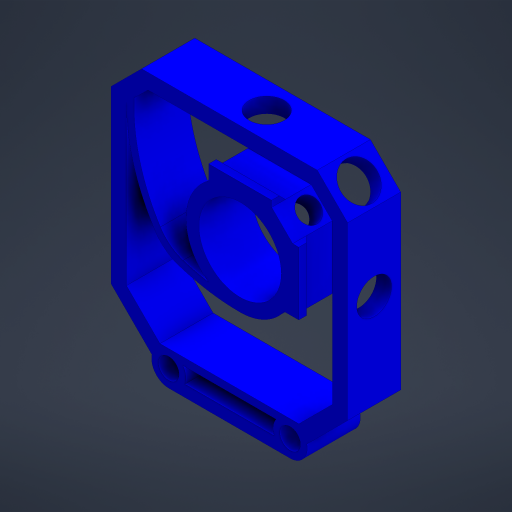
# Autodesk Inventor part: SM05 Lense Holder (V5)
Saved by Autodesk Inventor 2023.4 (Build 274418000, 418)
## iProperties
Created: 2022-07-25
Part Number: SM05 Lense Holder (V5)
Material: Generic
Document SubType Name: Modeling
Designer: xSibe
Density: 1 g/cm^3
Appearance: Plastic Blue
Author: xSibe
Autodesk Inventor part; units mm, degrees
ref_plane "YZ Plane" through (0, 0, 0) normal (1, 0, 0) x (0, 1, 0)
ref_plane "XZ Plane" through (0, 0, 0) normal (0, 1, 0) x (-1, 0, 0)
sketch "Sketch1" plane through (0, 0, 0) normal (0, 0, 1) x (1, 0, 0)
  circle A0 centre (139.6, 3.85) radius 2.8125
  circle A1 centre (159.6, 3.85) radius 2.8125
  line L0 (159.6, 1.0375) -> (139.6, 1.0375)
  line L1 (132.55, 24.9) -> (166.65, 24.9)
  line L2 (149.6, 24.9) -> (151.367767, 26.667767)
  line L3 (149.6, 24.9) -> (152.1, 24.9) construction
  circle A2 centre (151.367767, 26.667767) radius 6.78375
  circle A3 centre (151.367767, 26.667767) radius 6.10875
  circle A4 centre (151.367767, 26.667767) radius 8.90875
  line L4 (151.367767, 26.667767) -> (151.367767, 35.576517)
  line L5 (151.367767, 35.576517) -> (151.367767, 35.076517)
  line L6 (146.180267, 33.826517) -> (156.555267, 33.826517)
  line L7 (156.555267, 33.826517) -> (156.555267, 36.326517)
  line L8 (156.555267, 36.326517) -> (146.180267, 36.326517)
  line L9 (146.180267, 36.326517) -> (146.180267, 33.826517)
  line L10 (146.180267, 33.826517) -> (156.555267, 36.326517) construction
  line L11 (156.555267, 33.826517) -> (146.180267, 36.326517) construction
  line L12 (151.367767, 26.667767) -> (157.667204, 32.967204)
  line L13 (157.667204, 32.967204) -> (157.225263, 32.525263)
  line L14 (160.05369, 31.818156) -> (156.518156, 35.35369)
  line L15 (156.518156, 35.35369) -> (154.396836, 33.23237)
  line L16 (154.396836, 33.23237) -> (157.93237, 29.696836)
  line L17 (157.93237, 29.696836) -> (160.05369, 31.818156)
  line L18 (160.05369, 31.818156) -> (154.396836, 33.23237) construction
  line L19 (156.518156, 35.35369) -> (157.93237, 29.696836) construction
  line L20 (160.05369, 31.818156) -> (165.05369, 31.818156) construction
  line L21 (158.526517, 21.480267) -> (158.526517, 31.855267)
  line L22 (158.526517, 31.855267) -> (161.026517, 31.855267)
  line L23 (161.026517, 31.855267) -> (161.026517, 21.480267)
  line L24 (161.026517, 21.480267) -> (158.526517, 21.480267)
  line L25 (151.367767, 35.576517) -> (151.367767, 37.576517)
  line L26 (161.026517, 26.667767) -> (163.026517, 26.667767)
  line L27 (139.382233, 5.432233) -> (159.817767, 5.432233)
  line L28 (169.067767, 14.682233) -> (169.067767, 39.367767)
  line L29 (164.067767, 44.367767) -> (135.132233, 44.367767)
  line L30 (130.132233, 39.367767) -> (130.132233, 14.682233)
  line L31 (130.132233, 5.432233) -> (169.067767, 44.367767) construction
  line L32 (169.067767, 5.432233) -> (130.132233, 44.367767) construction
  line L33 (139.382233, 5.432233) -> (130.132233, 14.682233)
  line L34 (159.817767, 5.432233) -> (169.067767, 14.682233)
  line L35 (164.067767, 44.367767) -> (169.067767, 39.367767)
  line L36 (135.132233, 44.367767) -> (130.132233, 39.367767)
  line L37 (134.096699, 46.867767) -> (127.632233, 40.403301)
  line L38 (127.632233, 40.403301) -> (127.632233, 13.646699)
  line L39 (127.632233, 13.646699) -> (138.346699, 2.932233)
  line L40 (138.346699, 2.932233) -> (160.853301, 2.932233)
  line L41 (160.853301, 2.932233) -> (171.567767, 13.646699)
  line L42 (171.567767, 13.646699) -> (171.567767, 40.403301)
  line L43 (171.567767, 40.403301) -> (165.103301, 46.867767)
  line L44 (165.103301, 46.867767) -> (134.096699, 46.867767)
  line L45 (136.167767, 41.867767) -> (132.632233, 38.332233)
  line L46 (132.632233, 38.332233) -> (132.632233, 15.717767)
  line L47 (132.632233, 15.717767) -> (140.417767, 7.932233)
  line L48 (140.417767, 7.932233) -> (158.782233, 7.932233)
  line L49 (158.782233, 7.932233) -> (166.567767, 15.717767)
  line L50 (166.567767, 15.717767) -> (166.567767, 38.332233)
  line L51 (166.567767, 38.332233) -> (163.032233, 41.867767)
  line L52 (163.032233, 41.867767) -> (136.167767, 41.867767)
  line L53 (130.132233, 14.682233) -> (130.132233, 11.146699)
  line L54 (169.067767, 14.682233) -> (169.067767, 11.146699)
  circle A5 centre (139.6, 3.85) radius 1.705
  circle A6 centre (159.6, 3.85) radius 1.705
  line L55 (151.367767, 17.759017) -> (138.867767, 17.759017)
  line L56 (138.867767, 17.759017) -> (138.867767, 20.259017)
  arc A7 (138.867767, 20.259017) -> (151.367767, 17.759017) centre (151.367767, 50.259017) ccw
  arc A8 (132.632233, 38.332233) -> (138.867767, 20.259017) centre (161.941914, 38.332233) ccw
  arc A9 (133.911405, 39.611405) -> (139.651699, 21.288407) centre (161.941914, 38.332233) ccw
  arc A10 (139.651699, 21.288407) -> (146.148582, 19.447938) centre (151.367767, 50.259017) ccw
  line L57 (138.867767, 20.259017) -> (137.411533, 22.291105)
  line L58 (139.651699, 21.288407) -> (138.223144, 23.340048)
  arc A11 (137.411533, 22.291105) -> (141.173712, 19.399152) centre (143.428852, 26.226005) ccw
  arc A12 (138.223144, 23.340048) -> (141.966404, 20.45672) centre (144.034782, 27.013474) ccw
  line L59 (132.55, 7.7) -> (132.55, 42.1)
  line L60 (166.65, 7.7) -> (166.65, 42.1)
  circle A13 centre (139.6, 3.85) radius 1.5625
  circle A14 centre (159.6, 3.85) radius 1.5625
  line L61 (138.151966, 6.6625) -> (161.048034, 6.6625)
  line L62 (139.6, 5.555) -> (159.6, 5.555)
  line L63 (139.6, 2.145) -> (159.6, 2.145)
  line L64 (132.632233, 15.717767) -> (132.632233, 12.182233)
  line L65 (166.567767, 15.717767) -> (166.567767, 12.182233)
  point P0 (156.941455, 2.932233)
  point P1 (142.258545, 2.932233)
  point P2 (138.414176, 6.40029)
  point P3 (160.785824, 6.40029)
  point P4 (146.180267, 33.910396)
  point P5 (158.610396, 21.480267)
  point P6 (158.610396, 31.855267)
  point P7 (159.181848, 30.946314)
  point P8 (155.646314, 34.481848)
  point P9 (156.555267, 33.910396)
  point P10 (162.351875, 4.430808)
  point P11 (136.848125, 4.430808)
  point P12 (154.990983, 33.826517)
  point P13 (-2.842005, 34.542767)
  point P14 (9.642767, 22.057995)
  point P15 (158.526517, 30.290983)
  point P16 (10.676517, 26.667767)
  point P17 (160.016579, 31.855267)
  point P18 (9.642767, 31.277539)
  point P19 (6.377539, 34.542767)
  point P20 (1.767767, 35.576517)
  point P21 (156.555267, 35.316579)
  point P22 (8.067204, 32.967204)
  point P23 (166.567767, 24.9)
  point P24 (132.632233, 24.9)
  point P25 (160.099366, 24.9)
  point P26 (142.636168, 24.9)
  point P27 (157.27477, 5.432233)
  point P28 (141.92523, 5.432233)
  point P29 (156.164603, 31.464603)
  point P30 (138.573172, 22.837349)
  dimension "d2" = 2.5
  dimension "d3" = 45
  dimension "d4" = 13.5675
  dimension "d5" = 0.675
  dimension "d6" = 2.125
  dimension "d7" = 0.5
  dimension "d8" = 10.375
  dimension "d9" = 2.5
  dimension "d10" = 0.625
  dimension "d11" = 5
  dimension "d12" = 135
  dimension "d13" = 3
  dimension "d14" = 2
  dimension "d15" = 2
  dimension "d16" = 38.93553
  dimension "d17" = 38.93553
  dimension "d18" = 9.25
  dimension "d19" = 9.25
  dimension "d20" = 9.25
  dimension "d21" = 9.25
  dimension "d22" = 5
  dimension "d23" = 5
  dimension "d24" = 5
  dimension "d25" = 5
  dimension "d26" = 2.5
  dimension "d46" = 2.5
  dimension "d50" = 12.5
  dimension "d51" = 2.5
  dimension "d52" = 1.25
  dimension "d53" = 2.5
  dimension "d54" = 2.5
  dimension "d55" = 0.1425
  dimension "d56" = 0.1425
  dimension "d57" = 1.25
  dimension "d58" = 1.25
  constraints: 128 end point, 24 point on circle, 19 point on line, 11 centre point, 11 parallel, 11 tangent, 10 horizontal, 10 midpoint, 8 perpendicular, 4 symmetric about line, 3 coincident, 2 equal length, 2 vertical, 1 collinear, 21 other
  measures "d2" distance of L2.start L2.end
  measures "d3" angle of L3 L2
  measures "d4" diameter of A2
  measures "d5" radial gap between concentric circles of A2 A3
  measures "d6" radial gap between concentric circles of A2 A4
  measures "d7" distance of L4.end L5.end
  measures "d8" distance of L8.end L7.end
  measures "d9" distance of L7.end L6.end
  measures "d10" distance of L12.end L13.end
  measures "d11" distance of L14.start L14.end
  measures "d12" angle of L20 L14
  measures "d13" distance of L15.end L14.end
  measures "d14" distance of L4.end L25.end
  measures "d15" distance of L26.start L26.end
  measures "d16" distance of L31.end L32.end
  measures "d17" distance of L32.end L31.start
  measures "d18" distance of L27.start L31.start
  measures "d19" distance of L30.end L31.start
  measures "d20" distance of L27.end L32.start
  measures "d21" distance of L28.start L32.start
  measures "d22" distance of L29.start L31.end
  measures "d23" distance of L28.end L31.end
  measures "d24" distance of L29.end L32.end
  measures "d25" distance of L30.start L32.end
  measures "d26" distance between parallel lines of L29 L44
  measures "d46" distance between parallel lines of L29 L52
  measures "d50" distance of L55.start L55.end
  measures "d51" distance of L55.end L56.end
  measures "d52" radial gap between concentric circles of A8 A9
  measures "d53" distance of L56.end L57.end
  measures "d54" distance of L58.start L58.end
  measures "d55" radial gap between concentric circles of A5 A13
  measures "d56" radial gap between concentric circles of A6 A14
extrude "Extrusion1" add sketch "Sketch1" along normal mid plane 8.75 contours A0 L40 A5 L27 | L27 A5 L62 A0 | A0 L62 A1 L27 | L40 A1 L63 A0 | A0 L63 A5 L40 | L62 A5 L33 A0 | A0 L61 A1 L62 | L27 A6 L40 A1 | A1 L62 A6 L27 | L63 A1 L0 A0 | A0 L39 A5 L63 | L40 A6 L63 A1 | A0 L33 L61 | A1 L34 A6 L62 | L63 A6 L41 A1 | L33 A5 L39 A0 | A0 L39 L59 L33 | L61 L34 A1 | L33 L59 L1 L46 L64 | L34 L60 L41 A1 | A1 L41 A6 L34 | L39 L53 L33 L59 | L33 L30 L36 L59 | L65 L50 L1 L60 L34 | L59 L36 L29 L35 L60 L1 L50 L51 L52 L45 L46 | L60 L34 L54 L41 | L60 L35 L28 L34 | A8 L45 A9 L1 | L1 A9 A10 A4 A7 A11 L57 A8 | L57 A11 | L23 L24 A4 L1 | L1 A4 L17 L14 L22 L23 | A4 L9 L6 L4 A2 L1 | L1 A2 L21 L24 A4 | A12 L58 A9 | A4 L24 L21 L1 | L1 L21 L17 A4 | L9 L8 L25 A4 | A4 L4 L6 L9 | L58 A12 A10 | L1 A2 L16 L17 L21 | L4 L6 L15 L16 A2 | L25 L8 L7 L14 L15 A4 | A4 L15 L6 L4 | L21 L22 A4 L17 | L17 L16 L12 A4 L22 L21 | A4 L22 L14 L17 | L22 A4 L7 L14 | L16 L15 L6 L7 A4 L12 | L15 L14 L7 A4 | A4 L7 L6 L15
sketch "Sketch2" plane through (0, 0, 0) normal (0, 0, 1) x (1, 0, 0)
  circle A0 centre (151.367767, 26.667767) radius 6.78375
  circle A1 centre (151.367767, 26.667767) radius 5.90875
  point P0 (0, 0)
  dimension "d30" = 0.875
  constraints: 1 centre point
  measures "d30" radial gap between concentric circles of A0 A1
extrude "Extrusion2" [suppressed]
sketch "Sketch3" plane through (169.067767, 13.646699, -4.375) normal (1, 0, 0) x (0, 0, -1)
  line L0 (0, 7.833568) -> (-8.75, 7.833568)
  line L1 (0, 18.208568) -> (0, 7.833568)
  line L2 (0, 18.208568) -> (-8.75, 18.208568)
  line L3 (-8.75, 7.833568) -> (-8.75, 18.208568)
  line L4 (-4.375, 18.208568) -> (-4.375, 7.833568)
  circle A0 centre (-4.375, 13.021068) radius 2.875
  point P0 (-4.375, -13.646699)
  dimension "d33" = 5.75
  constraints: 3 midpoint, 2 end point, 1 centre point
  measures "d33" diameter of A0
extrude "Extrusion3" cut sketch "Sketch3" against normal up to surface (2.5 mm away) contours A0 L4 | L4 A0
sketch "Sketch4" plane through (159.448814, 31.855267, -4.375) normal (0, 1, 0) x (1, 0, 0)
  line L0 (1.577703, 0) -> (1.577703, -8.75)
  line L1 (0.567765, 0) -> (1.577703, 0)
  line L2 (1.577703, -8.75) -> (0.567765, -8.75)
  line L3 (1.577703, -8.75) -> (0.567765, -8.75)
  line L4 (0.567765, -8.75) -> (0.567765, -7.5)
  line L5 (0.567765, -7.5) -> (1.577703, -7.5)
  line L6 (1.577703, -7.5) -> (1.577703, -8.75)
  line L7 (1.577703, -7.5) -> (0.567765, -6.490062)
  line L8 (1.577703, -7.5) -> (3.005971, -7.5) construction
  line L9 (0.567765, -4.375) -> (1.577703, -4.375)
  line L10 (1.577703, -1.25) -> (0.567765, -2.259938)
  line L11 (0.567765, 0) -> (0.567765, -8.75)
  point P0 (-159.448814, -4.375)
  point P1 (1.577703, -1.25)
  point P2 (1.577703, -7.5)
  point P3 (0.567765, -8.75)
  point P4 (0.567765, -6.740062)
  point P5 (0.567765, -2.259938)
  dimension "d36" = 1.25
  dimension "d37" = 135
  constraints: 16 end point, 3 horizontal, 2 midpoint, 2 parallel, 2 symmetric about line, 1 equal length, 1 perpendicular, 1 point on line
  measures "d36" distance of L2.end L4.end
  measures "d37" angle of L8 L7
extrude "Extrusion4" cut sketch "Sketch4" against normal up to surface (10.375 mm away) contours L0 L9 L11 L10 | L0 L7 L11 L9
ref_plane "Work Plane1" through (161.026517, 36.326517, 4.375) normal (0.7071068, -0.7071068, 0) x (0, 0, -1)
mirror "Mirror1" about plane through (161.026517, 36.326517, 4.375) normal (0.7071068, -0.7071068, 0) of "Extrusion3", "Extrusion4"
sketch "Sketch5" plane through (169.8, 38.635534, 4.375) normal (0.7071068, 0.7071068, 0) x (0.7071068, -0.7071068, 0)
  circle A0 centre (-4.571068, 4.375) radius 1.875
  line L0 (-7.018585, 4.375) -> (-2.123551, 4.375)
  circle A1 centre (-4.571068, 4.375) radius 3
  line L1 (-7.018585, 0) -> (-7.018585, 2.259938)
  line L2 (-2.123551, 0) -> (-7.018585, 0)
  line L3 (-2.123551, 8.75) -> (-2.123551, 6.490062)
  line L4 (-7.018585, 8.75) -> (-2.123551, 8.75)
  line L5 (-7.018585, 6.490062) -> (-7.018585, 8.75)
  line L6 (-7.018585, 2.259938) -> (-7.018585, 6.490062)
  line L7 (-2.123551, 2.259938) -> (-2.123551, 0)
  line L8 (-2.123551, 6.490062) -> (-2.123551, 2.259938)
  point P0 (-92.747283, 4.375)
  dimension "d28" = 8.75
  dimension "d40" = 3.75
  dimension "d41" = 6
  constraints: 3 midpoint, 2 centre point, 2 end point, 1 coincident
  measures "d40" diameter of A0
  measures "d41" diameter of A1
extrude "Extrusion5" cut sketch "Sketch5" against normal blind 5 contours L0 A0 | L0 L8 A1 L6 A0 | A0 L0 L6 A1 L8 | A0 L0 | L8 A1 | L6 A1
extrude "Extrusion6" cut sketch "Sketch5" against normal up to next from surface at -11.712296 contours L0 A0 | A0 L0
equation "\"d19\" = d18"
equation "\"d20\" = d18"
equation "\"d21\" = d20"
equation "\"d23\" = d22"
equation "\"d24\" = d22"
equation "\"d25\" = d24"
body "Solid1"
